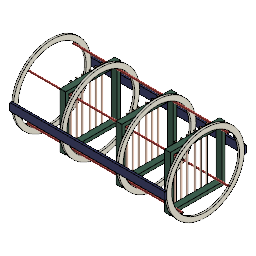
IonenAntrieb v3 (Autodesk Fusion 360 design; units mm, degrees)
Autodesk Fusion 360 part; units mm, degrees
note: some values were not read from the file. Chosen so that the rebuilt part matches the saved one: which bodies a step acts on; which face or edge a step refers to. Set by a fixed rule: which sketch regions a step uses.
sketch "Skizze2" plane through (0, 0, 0) normal (0, 0, 1) x (1, 0, 0)
  line L0 (200, -25) -> (-200, -25)
  line L1 (-200, -25) -> (-200, 25)
  line L2 (-200, 25) -> (200, 25)
  line L3 (200, 25) -> (200, -25)
  line L4 (200, -25) -> (-200, 25) construction
  line L5 (-200, -25) -> (200, 25) construction
  line L6 (100, -25) -> (-100, -25)
  line L7 (-100, -25) -> (-100, 25)
  line L8 (-100, 25) -> (100, 25)
  line L9 (100, 25) -> (100, -25)
  line L10 (100, -25) -> (-100, 25) construction
  line L11 (-100, -25) -> (100, 25) construction
  dimension "d4" = 400
  dimension "d5" = 50
  dimension "d6" = 200
  dimension "d7" = 50
  constraint horizontal L0
  constraint perpendicular L0 L1
  constraint parallel L0 L2
  constraint parallel L1 L3
  constraint coincident L4 origin
  constraint coincident L5 origin
  constraint horizontal L6
  constraint perpendicular L6 L7
  constraint parallel L6 L8
  constraint parallel L7 L9
  constraint coincident L10 origin
  constraint coincident L11 origin
  measures "d4" distance of L1.end L2.end
  measures "d5" distance of L0.end L1.end
  measures "d6" distance of L7.end L8.end
  measures "d7" distance of L6.end L7.end
sketch "Skizze3" plane through (0, 0, 0) normal (0, 0, 1) x (1, 0, 0)
  line L0 (75, -25) -> (-75, -25)
  line L1 (-75, -25) -> (-75, 25)
  line L2 (-75, 25) -> (75, 25)
  line L3 (75, 25) -> (75, -25)
  line L4 (75, -25) -> (-75, 25) construction
  line L5 (-75, -25) -> (75, 25) construction
  dimension "d10" = 150
  dimension "d11" = 50
  constraint horizontal L0
  constraint perpendicular L0 L1
  constraint parallel L0 L2
  constraint parallel L1 L3
  constraint coincident L4 origin
  constraint coincident L5 origin
  measures "d10" distance of L1.end L2.end
  measures "d11" distance of L0.start L2.end
sketch "Skizze4" plane through (200, 0, 0) normal (1, 0, 0) x (0, 1, 0)
  line L0 (-25, 0) -> (25, 0)
  line L1 (25, 0) -> (25, 5)
  line L2 (25, 5) -> (-25, 5)
  line L3 (-25, 5) -> (-25, 0)
  circle A0 centre (0, 0) radius 100
  dimension "d14" = 200
  constraint coincident A0.centre origin
  measures "d14" diameter of A0
sketch "Skizze5" plane through (75, 0, 0) normal (1, 0, 0) x (0, 1, 0)
  line L0 (25, 0) -> (25, 10)
  line L1 (25, 10) -> (-25, 10)
  line L2 (-25, 10) -> (-25, 0)
  circle A0 centre (0, 0) radius 100
  line L3 (-25, 0) -> (25, 0)
  dimension "d15" = 200
  constraint coincident A0.centre origin
  measures "d15" diameter of A0
sketch "Skizze6" plane through (-200, 0, 0) normal (-1, 0, 0) x (0, -1, 0)
  line L0 (-25, 0) -> (25, 0)
  line L1 (25, 0) -> (25, 5)
  line L2 (25, 5) -> (-25, 5)
  line L3 (-25, 5) -> (-25, 0)
  circle A0 centre (0, 0) radius 100
  dimension "d16" = 200
  constraint coincident A0.centre origin
  measures "d16" diameter of A0
sketch "Skizze7" plane through (-75, 0, 0) normal (-1, 0, 0) x (0, -1, 0)
  line L0 (-25, 0) -> (25, 0)
  line L1 (25, 0) -> (25, 10)
  line L2 (25, 10) -> (-25, 10)
  line L3 (-25, 10) -> (-25, 0)
  circle A0 centre (0, 0) radius 100
  dimension "d17" = 200
  constraint coincident A0.centre origin
  measures "d17" diameter of A0
extrude "Extrusion4" add sketch "Skizze4" along normal blind 0 and the other way blind 5 contours L0 L1 L2 L3 | A0 makes body 1
extrude "Extrusion5" add sketch "Skizze5" along normal blind 0 and the other way blind 5 separate body contours L0 L1 L2 L3 | A0 makes body 2
extrude "Extrusion6" add sketch "Skizze7" along normal blind 0 and the other way blind 5 separate body contours L0 L1 L2 L3 | A0 makes body 3
extrude "Extrusion7" add sketch "Skizze6" along normal blind 0 and the other way blind 5 separate body contours L0 L1 L2 L3 | A0 makes body 4
hole "Bohrung1" at (-200, 0, 0) direction (1, 0, 0) diameter 175 depth 1000 tip angle 118 bodies 1 2 3 4
sketch "Skizze14" plane through (200, 0, 0) normal (1, 0, 0) x (0, 1, 0)
  circle A0 centre (0, 0) radius 87.5
  circle A1 centre (0, 0) radius 100
  line L0 (70.7107, 70.7107) -> (-70.7107, 70.7107)
  line L1 (-70.7107, 70.7107) -> (-70.7107, -70.7107)
  line L2 (-70.7107, -70.7107) -> (70.7107, -70.7107)
  line L3 (70.7107, -70.7107) -> (70.7107, 70.7107)
  line L4 (70.7107, 70.7107) -> (-70.7107, -70.7107) construction
  line L5 (-70.7107, 70.7107) -> (70.7107, -70.7107) construction
  dimension "d66" = 200
  dimension "d67" = 200
  dimension "d68" = 90
  dimension "d69" = 90
  constraint horizontal L0
  constraint perpendicular L0 L1
  constraint parallel L0 L2
  constraint parallel L1 L3
  constraint coincident L4 A0.centre
  constraint coincident L5 A0.centre
  constraint coincident A0.centre A1.centre
  measures "d66" distance of L0.start L1.end
  measures "d67" distance of L0.end L2.end
  measures "d68" angle of L4 L5
  measures "d69" angle of L4 L5
extrude "Extrusion11" add sketch "Skizze14" along normal blind -20 and the other way blind 305 separate body contours A0 L0 L1 L2 L3 | A0 L0 L3 | A0 L2 L3 | A0 L0 L1 | A0 L1 L2 makes body 5
sketch "Skizze15" plane through (200, 0, 0) normal (1, 0, 0) x (0, 1, 0)
  circle A0 centre (0, 0) radius 87.5
  circle A1 centre (0, 0) radius 100
  line L0 (61.8718, 61.8718) -> (-61.8718, 61.8718)
  line L1 (-61.8718, 61.8718) -> (-61.8718, -61.8718)
  line L2 (-61.8718, -61.8718) -> (61.8718, -61.8718)
  line L3 (61.8718, -61.8718) -> (61.8718, 61.8718)
  line L4 (61.8718, 61.8718) -> (-61.8718, -61.8718) construction
  line L5 (-61.8718, 61.8718) -> (61.8718, -61.8718) construction
  dimension "d77" = 90
  dimension "d78" = 175
  constraint horizontal L0
  constraint perpendicular L0 L1
  constraint parallel L0 L2
  constraint parallel L1 L3
  constraint coincident L4 A0.centre
  constraint coincident L5 A0.centre
  constraint coincident A0.centre A1.centre
  measures "d77" angle of L4 L5
  measures "d78" distance of L0.start L1.end
extrude "Extrusion12" cut sketch "Skizze15" along normal blind 0 and the other way blind 370 contours L0 L1 L2 L3 bodies 5
sketch "Skizze16" plane through (0, 70.7107, 0) normal (0, 1, 0) x (-1, 0, 0)
  line L0 (-180, 70.7107) -> (-180, -70.7107)
  line L1 (105, -70.7107) -> (105, 70.7107)
  line L2 (-160, 80) -> (-75, 80)
  line L3 (-75, 80) -> (-75, -80)
  line L4 (-75, -80) -> (-160, -80)
  line L5 (-160, -80) -> (-160, 80)
  line L6 (-180, -70.7107) -> (105, -70.7107)
  line L7 (105, 70.7107) -> (-180, 70.7107)
  dimension "d83" = 85
  dimension "d84" = 160
  dimension "d85" = 90
  constraint horizontal L2
  constraint vertical L3
  constraint horizontal L4
  constraint vertical L5
  measures "d83" distance of L3.end L4.end
  measures "d84" distance of L2.start L4.end
  measures "d85" angle of L2 L3
extrude "Extrusion13" cut sketch "Skizze16" against normal blind 430 contours L3 L5 L6 L7 | L2 L3 L5 L7 | L3 L4 L5 L6 bodies 5 makes body 6 at (180, 67.7644, -20.6239)
sketch "Skizze17" plane through (0, 70.7107, 0) normal (0, 1, 0) x (-1, 0, 0)
  line L0 (-160, -70.7107) -> (-160, 70.7107)
  line L1 (-180, 70.7107) -> (-180, -70.7107)
  line L2 (-160, -75) -> (-165, -75)
  line L3 (-165, -75) -> (-165, 75)
  line L4 (-165, 75) -> (-160, 75)
  line L5 (-160, 75) -> (-160, -75)
  line L6 (-160, 70.7107) -> (-180, 70.7107)
  line L7 (-180, -70.7107) -> (-160, -70.7107)
  dimension "d88" = 20
  dimension "d89" = 5
  dimension "d90" = 150
  constraint horizontal L2
  constraint vertical L3
  constraint horizontal L4
  constraint vertical L5
  measures "d88" distance of L0 L1
  measures "d89" distance of L2.start L2.end
  measures "d90" distance of L2.start L4.end
extrude "Extrusion14" cut sketch "Skizze17" against normal blind 300 contours L0 L3 L5 L6 L7 | L2 L3 L5 L7 | L3 L4 L5 L6 bodies 6
sketch "Skizze18" plane through (0, 70.7107, 0) normal (0, 1, 0) x (-1, 0, 0)
  line L0 (-75, 70.7107) -> (-75, -70.7107)
  line L1 (105, -70.7107) -> (105, 70.7107)
  line L2 (-70, -75) -> (-55, -75)
  line L3 (-55, -75) -> (-55, 95)
  line L4 (-55, 95) -> (-70, 95)
  line L5 (-70, 95) -> (-70, -75)
  line L6 (-75, -70.7107) -> (105, -70.7107)
  line L7 (105, 70.7107) -> (-75, 70.7107)
  dimension "d93" = 15
  dimension "d94" = 170
  constraint horizontal L2
  constraint vertical L3
  constraint horizontal L4
  constraint vertical L5
  measures "d93" distance of L2.start L2.end
  measures "d94" distance of L2.start L4.end
extrude "Extrusion15" cut sketch "Skizze18" against normal blind 440 contours L3 L5 L6 L7 | L3 L4 L5 L7 | L2 L3 L5 L6 bodies 5 makes body 7 at (75, -20.6239, 67.7644)
sketch "Skizze19" plane through (0, -70.7107, 0) normal (0, -1, 0) x (1, 0, 0)
  line L0 (55, -70.7107) -> (55, 70.7107)
  line L1 (-105, 70.7107) -> (-105, -70.7107)
  line L2 (-75, -75) -> (-90, -75)
  line L3 (-90, -75) -> (-90, 1425)
  line L4 (-90, 1425) -> (-75, 1425)
  line L5 (-75, 1425) -> (-75, -75)
  line L6 (180, -51.5388) -> (165, -51.5388)
  line L7 (55, 70.7107) -> (-105, 70.7107)
  line L8 (-105, -70.7107) -> (55, -70.7107)
  dimension "d97" = 15
  dimension "d98" = 1500
  dimension "d99" = 15
  constraint horizontal L2
  constraint vertical L3
  constraint horizontal L4
  constraint vertical L5
  measures "d97" distance of L2.start L2.end
  measures "d98" distance of L2.start L4.end
  measures "d99" distance of L6.start L6.end
extrude "Extrusion16" cut sketch "Skizze19" against normal blind 170 contours L3 L5 L7 L8 | L2 L3 L5 L8 | L3 L4 L5 L7 bodies 5 makes body 8 at (11.6667, -70.7107, 23.5702)
sketch "Skizze21" plane through (0, 70.7107, 0) normal (0, 1, 0) x (-1, 0, 0)
  line L0 (75, -70.7107) -> (75, 70.7107)
  line L1 (-55, 70.7107) -> (-55, -70.7107)
  line L2 (-55, 75) -> (-40, 75)
  line L3 (-40, 75) -> (-40, -75)
  line L4 (-40, -75) -> (-55, -75)
  line L5 (-55, -75) -> (-55, 75)
  line L6 (-90, 80) -> (-65, 80)
  line L7 (-65, 80) -> (-65, -75)
  line L8 (-65, -75) -> (-90, -75)
  line L9 (-90, -75) -> (-90, 80)
  line L10 (-40, 75) -> (78.1295, 75)
  line L11 (78.1295, 75) -> (78.1295, -86.3488)
  line L12 (78.1295, -86.3488) -> (-40, -86.3488)
  line L13 (-40, -86.3488) -> (-40, 75)
  line L14 (75, 70.7107) -> (-55, 70.7107)
  line L15 (-55, -70.7107) -> (75, -70.7107)
  dimension "d102" = 15
  dimension "d103" = 150
  constraint horizontal L2
  constraint vertical L3
  constraint horizontal L4
  constraint vertical L5
  constraint horizontal L6
  constraint vertical L7
  constraint horizontal L8
  constraint vertical L9
  constraint horizontal L10
  constraint vertical L11
  constraint horizontal L12
  constraint vertical L13
  measures "d102" distance of L2.start L2.end
  measures "d103" distance of L2.start L4.end
extrude "Extrusion17" cut sketch "Skizze21" against normal blind 355 contours L0 L3 L13 L14 L15 | L0 L3 L10 L11 L12 L13 L14 L15 bodies 8
sketch "Skizze23" plane through (0, 70.7107, 0) normal (0, 1, 0) x (-1, 0, 0)
  line L0 (-70, -70.7107) -> (-70, 70.7107)
  line L1 (-75, 70.7107) -> (-75, -70.7107)
  line L2 (-85, 75) -> (-60, 75)
  line L3 (-60, 75) -> (-60, -75)
  line L4 (-60, -75) -> (-85, -75)
  line L5 (-85, -75) -> (-85, 75)
  line L6 (-70, 70.7107) -> (-75, 70.7107)
  line L7 (-75, -70.7107) -> (-70, -70.7107)
  constraint horizontal L2
  constraint vertical L3
  constraint horizontal L4
  constraint vertical L5
extrude "Extrusion19" cut sketch "Skizze23" against normal blind 420 contours L0 L1 L6 L7 | L2 L3 L4 L5 bodies 7
sketch "Skizze26" plane through (180, 0, 0) normal (1, 0, 0) x (0, 1, 0)
  line L0 (-61.8718, 61.8718) -> (61.8718, 61.8718)
  line L1 (61.8718, 61.8718) -> (61.8718, -61.8718)
  line L2 (61.8718, -61.8718) -> (-61.8718, -61.8718)
  line L3 (-61.8718, -61.8718) -> (-61.8718, 61.8718)
  line L4 (70.7107, -70.7107) -> (70.7107, 70.7107)
  line L5 (70.7107, 70.7107) -> (-70.7107, 70.7107)
  line L6 (-70.7107, 70.7107) -> (-70.7107, -70.7107)
  line L7 (-70.7107, -70.7107) -> (70.7107, -70.7107)
  line L8 (-61.8718, -61.8718) -> (-56.8718, -61.8718)
  line L9 (-56.8718, -61.8718) -> (-56.8718, -56.8718)
  line L10 (-56.8718, -56.8718) -> (-61.8718, -56.8718)
  line L11 (-61.8718, -56.8718) -> (-61.8718, -61.8718)
  circle A0 centre (-59.3718, -59.3718) radius 2.5
  line L12 (61.8718, -61.8718) -> (56.8718, -61.8718)
  line L13 (56.8718, -61.8718) -> (56.8718, -56.8718)
  line L14 (56.8718, -56.8718) -> (61.8718, -56.8718)
  line L15 (61.8718, -56.8718) -> (61.8718, -61.8718)
  circle A1 centre (59.3718, -59.3718) radius 2.5
  line L16 (61.8718, 61.8718) -> (56.8718, 61.8718)
  line L17 (56.8718, 61.8718) -> (56.8718, 56.8718)
  line L18 (56.8718, 56.8718) -> (61.8718, 56.8718)
  line L19 (61.8718, 56.8718) -> (61.8718, 61.8718)
  circle A2 centre (59.3718, 59.3718) radius 2.5
  line L20 (-61.8718, 61.8718) -> (-56.8718, 61.8718)
  line L21 (-56.8718, 61.8718) -> (-56.8718, 56.8718)
  line L22 (-56.8718, 56.8718) -> (-61.8718, 56.8718)
  line L23 (-61.8718, 56.8718) -> (-61.8718, 61.8718)
  circle A3 centre (-59.3718, 59.3718) radius 2.5
  dimension "d111" = 5
  dimension "d112" = 5
  dimension "d113" = 5
  dimension "d114" = 2.5
  dimension "d115" = 5
  dimension "d116" = 5
  dimension "d117" = 5
  dimension "d118" = 5
  dimension "d119" = 5
  dimension "d120" = 5
  dimension "d121" = 5
  dimension "d122" = 5
  dimension "d123" = 5
  constraint horizontal L8
  constraint vertical L9
  constraint horizontal L10
  constraint vertical L11
  constraint coincident L2.end L3.start
  constraint tangent L10 A0
  constraint horizontal L12
  constraint vertical L13
  constraint horizontal L14
  constraint vertical L15
  constraint coincident L1.end L2.start
  constraint tangent L14 A1
  constraint horizontal L16
  constraint vertical L17
  constraint horizontal L18
  constraint vertical L19
  constraint coincident L0.end L1.start
  constraint tangent L16 A2
  constraint horizontal L20
  constraint vertical L21
  constraint horizontal L22
  constraint vertical L23
  constraint coincident L0.start L3.end
  constraint tangent L22 A3
  measures "d111" distance of L2.end L8.end
  measures "d112" distance of L2.end L10.end
  measures "d113" diameter of A0
  measures "d114" vertical distance of L2.end A0.centre
  measures "d115" distance of L1.end L12.end
  measures "d116" distance of L1.end L14.end
  measures "d117" diameter of A1
  measures "d118" distance of L0.end L16.end
  measures "d119" distance of L0.end L18.end
  measures "d120" diameter of A2
  measures "d121" distance of L0.start L20.end
  measures "d122" distance of L0.start L22.end
  measures "d123" diameter of A3
extrude "Extrusion20" add sketch "Skizze26" along normal blind 20 and the other way blind 380 separate body contours A3 | A2 | A0 | A1 makes body 9 at (66.6667, 60.3887, 61.6557) makes body 10 at (-73.3333, 61.8623, -59.5897) makes body 11 at (66.6667, -58.355, 61.6557) makes body 12 at (66.6667, -57.2068, -58.1218)
sketch "Skizze27" plane through (0, 0, 70.7107) normal (0, 0, 1) x (-1, 0, 0)
  line L0 (-165, -70.7107) -> (-165, 70.7107)
  line L1 (-165, 70.7107) -> (-180, 70.7107)
  line L2 (-180, 70.7107) -> (-180, -70.7107)
  line L3 (-180, -70.7107) -> (-165, -70.7107)
  circle A0 centre (-162.5, -9.991) radius 2.5
  circle A1 centre (-162.5, 10.0189) radius 2.5001
  circle A2 centre (-162.5, 24.9945) radius 2.5
  circle A3 centre (-162.5, -24.9732) radius 2.5001
  circle A4 centre (-162.5, 39.9853) radius 2.5
  circle A5 centre (-162.5, -39.9842) radius 2.5
  circle A6 centre (-37.5, 24.9945) radius 2.5
  circle A7 centre (-37.5, -39.9842) radius 2.5
  circle A8 centre (-37.5, -24.9732) radius 2.5001
  circle A9 centre (-37.5, 39.9853) radius 2.5
  circle A10 centre (-37.5, -9.991) radius 2.5
  circle A11 centre (-37.5, 10.0189) radius 2.5001
  circle A12 centre (107.5, 39.9853) radius 2.5
  circle A13 centre (107.5, -24.9732) radius 2.5001
  circle A14 centre (107.5, 10.0189) radius 2.5001
  circle A15 centre (107.5, 24.9945) radius 2.5
  circle A16 centre (107.5, -39.9842) radius 2.5
  circle A17 centre (107.5, -9.991) radius 2.5
extrude "Extrusion21" add sketch "Skizze27" along normal blind 0 and the other way blind 141.5 separate body contours A4 | A2 | A1 | A0 | A3 | A5 | A6 | A7 | A8 | A9 | A10 | A11 | A12 | A13 | A14 | A15 | A16 | A17 makes body 13 at (-105.5848, -8.4119, -23.6227) makes body 14 at (35.0773, -40.6022, -23.6227) makes body 15 at (35.0123, 25.2222, -23.6227) makes body 16 at (162.5623, 7.4918, -23.6227) makes body 17 at (162.5623, -42.4846, -23.6227) makes body 18 at (163.2963, 22.6033, -23.6227) makes body 19 at (35.0124, 10.2399, -23.6227) makes body 20 at (-105.5849, 41.5912, -23.6227) makes body 21 at (-108.5282, -27.2733, -23.6227) makes body 22 at (-109.2456, 8.2013, -23.6227) makes body 23 at (35.0124, -24.7456, -23.6227) makes body 24 at (39.9969, 40.1089, -23.6227) makes body 25 at (162.5623, -12.5182, -23.6227) makes body 26 at (161.0406, -27.0244, -23.6227) makes body 27 at (160.8458, 38.1098, 23.544) makes body 28 at (35.0124, -9.77, -23.6227) makes body 29 at (-107.4377, 22.4739, -23.6227) makes body 30 at (-105.1507, -40.8404, -23.6227)
sketch "Skizze28" plane through (200, 0, 0) normal (1, 0, 0) x (0, 1, 0)
  circle A0 centre (0, 0) radius 87.5
  circle A1 centre (0, 0) radius 100
  line L0 (-100, -10) -> (-87.5, -10)
  line L1 (-87.5, -10) -> (-87.5, 10)
  line L2 (-87.5, 10) -> (-100, 10)
  line L3 (-100, 10) -> (-100, -10)
  line L4 (-100, -10) -> (-87.5, 10) construction
  line L5 (-87.5, -10) -> (-100, 10) construction
  point P0 (-93.75, 0)
  dimension "d137" = 20
  dimension "d138" = 87.5
  dimension "d139" = 175
  constraint horizontal L0
  constraint perpendicular L0 L1
  constraint parallel L0 L2
  constraint parallel L1 L3
  constraint coincident L4 P0
  constraint coincident L5 P0
  measures "d137" distance of L0.start L2.end
  measures "d138" distance of A0.centre L1
  measures "d139" diameter of A0
extrude "Extrusion22" add sketch "Skizze28" against normal blind 5 contours A1 L0 L1 L2 | A1 L0 L3 | A1 L2 L3 picked at (-91.5924, -5.5576) bodies 1 2 3 4 5 6 8 9 10 11 12 13 14 15 16 17 18 19 20 21 22 23 24 25 26 27 28 29 30
sketch "Skizze31" plane through (0, -100, 0) normal (0, -1, 0) x (1, 0, 0)
  line L0 (195, 0) -> (195, -10)
  line L1 (195, -10) -> (200, -10)
  line L2 (200, -10) -> (200, 0)
  line L3 (200, 0) -> (200, 10)
  line L4 (200, 10) -> (195, 10)
  line L5 (195, 10) -> (195, 0)
  line L6 (200, -10) -> (-200, -10)
  line L7 (-200, -10) -> (-200, 10)
  line L8 (-200, 10) -> (200, 10)
  line L9 (200, 10) -> (200, -10)
  constraint horizontal L6
  constraint vertical L7
  constraint horizontal L8
  constraint vertical L9
  constraint coincident L1.end L2.start
extrude "Extrusion23" add sketch "Skizze31" along normal blind 5 separate body makes body 31
sketch "Skizze32" plane through (200, 0, 0) normal (1, 0, 0) x (0, 1, 0)
  arc A0 (-99.4987, -10) -> (-99.4987, 10) centre (0, 0) ccw
  line L0 (-99.4987, 10) -> (-100, 10)
  line L1 (-100, 10) -> (-100, 0)
  line L2 (-100, 0) -> (-100, -10)
  line L3 (-100, -10) -> (-99.4987, -10)
  circle A1 centre (0, 0) radius 87.5
  line L4 (100, -10) -> (88, -10)
  line L5 (88, -10) -> (88, 10)
  line L6 (88, 10) -> (100, 10)
  line L7 (100, 10) -> (100, -10)
  line L8 (100, -10) -> (88, 10) construction
  line L9 (88, -10) -> (100, 10) construction
  point P0 (94, 0)
  dimension "d142" = 12
  dimension "d143" = 20
  constraint horizontal L4
  constraint perpendicular L4 L5
  constraint parallel L4 L6
  constraint parallel L5 L7
  constraint coincident L8 P0
  constraint coincident L9 P0
  measures "d142" distance of L5.end L6.end
  measures "d143" distance of L4.end L5.end
extrude "Extrusion25" add sketch "Skizze32" against normal blind 5 contours A0 L4 L5 L6 | A0 L4 L7 | A0 L6 L7 bodies 1
sketch "Skizze33" plane through (0, 100, 0) normal (0, 1, 0) x (-1, 0, 0)
  line L0 (-195, -10) -> (-195, 10)
  line L1 (-195, 10) -> (-200, 10)
  line L2 (-200, 10) -> (-200, -10)
  line L3 (-200, -10) -> (-195, -10)
  line L4 (-200, 10) -> (200, 10)
  line L5 (200, 10) -> (200, -10)
  line L6 (200, -10) -> (-200, -10)
  line L7 (-200, -10) -> (-200, 10)
  constraint horizontal L4
  constraint vertical L5
  constraint horizontal L6
  constraint vertical L7
  constraint coincident L1.end L2.start
extrude "Extrusion26" add sketch "Skizze33" along normal blind 5 separate body makes body 32
